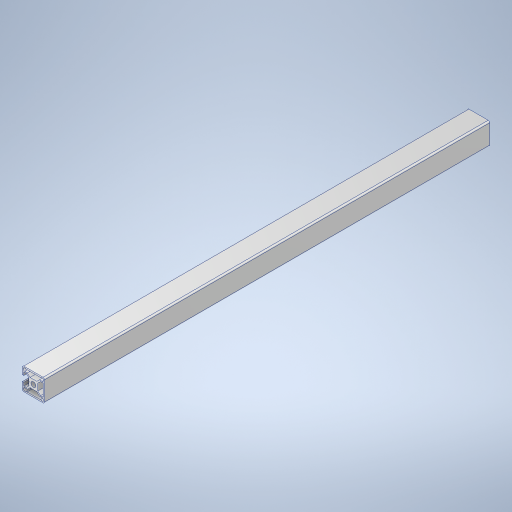
# Autodesk Inventor part: HFSC6-3030-600
Saved by Autodesk Inventor 2024 (Build 280153000, 153)
## iProperties
Category: PARTsolutions
Company: MISUMI
Created: 2024-12-02
Part Number: HFSC6-3030-600
Material: Aluminum 6061
Catalog Web Link: www.cadenas.de
Description: NEFSF6-3030, EFSF6-3030, EFSFB6-3030, HFSF6-3030, HFSFB6-3030, EFSH6-3030, HFSH6-3030, NEFST6-3030, EFST6-3030,  EFSTB6-3030, HFST6-3030, HFSTB6-3030, EFSC6-3030, HFSC6-3030-HFS6 Series Aluminum Extrusions 30 Square -1 Slot-
Vendor: MISUMI
Document SubType Name: Modeling
Designer: psAdmin
Manufacturer: MISUMI
Mass: 583.629 g
Surface Area: 2047.22 cm^2
Volume: 216.159 cm^3
Density: 2.7 g/cm^3
Appearance: Aluminum - Flat
PSOL_IDENT_0: {$CADENAS_DATA/23d-libs/misumi/metric/38_al_extrusions_blackets/6/hfsf6_3030.prj},748 {VTYP=3D},{NB=
PSOL_IDENT_1: HFSC6-3030-600},{LINA=HFSC6-3030-600},{NN=NEFSF6-3030, EFSF6-3030, EFSFB6-3030, HFSF6-3030, HFSFB6-3
PSOL_IDENT_2: 030, EFSH6-3030, HFSH6-3030, NEFST6-3030, EFST6-3030,  EFSTB6-3030, HFST6-3030, HFSTB6-3030, EFSC6-3
PSOL_IDENT_3: 030, HFSC6-3030},{DATE=31.01.2024 10:05:21},{GEOMDATE=26.07.2023 02:49:00},{VERSION=},{LINEID=190},{
PSOL_IDENT_4: WBVAR=L,ALT1,ALT2,ALT3,ALT4,ALT5,CP5,DL5,DR5,ALT6,ALT9,ALT10,ALT11,DD6SE,DD6,HP6,NHL6,DL6,NHR6,DR6,A
PSOL_IDENT_5: LT7,ALT8,NH9,AH,BH,CH,DH,EH,NH10,AV,BV,CV,DV,EV,NH11,AP,BP,CP,DP,EP,ALT12,ALT13,Z,NH12,XA,XB,XC,XD,X
PSOL_IDENT_6: E,NH13,YA,YB,YC,YD,YE,ALT14,HP14,DL14,DR14,ALT15,HP15,DL15,DR15,ALT16,HP16,DL16,DR16,ALT17,HQ17,JLP,
PSOL_IDENT_7: ALT20},{WBNUMERIC=L,DD6,NH9,AH,BH,CH,DH,EH,NH10,AV,BV,CV,DV,EV,NH11,AP,BP,CP,DP,EP,NH12,XA,XB,XC,XD,
PSOL_IDENT_8: XE,NH13,YA,YB,YC,YD,YE,HQ17,JLP}  {NB=HFSC6-3030-600},{LINA=HFSC6-3030-600},{KT=DUMMY},{PN=HFSC6-303
PSOL_IDENT_9: 0-600},{TPS=HFSC6-3030},{MAT=A6N01SS-T5 Aluminum Alloy},{ST=Clear Anodize},{FRMW=30},{FRMH=30},{FRD=
PSOL_IDENT_10: 6.8},{L=600.0},{MASS=0.97},{SA=361},{LX=2.99x10^4},{LY=3.24x10^4},{ALT1=},{M1=0},{DALT1=4.2},{DPL1=0
PSOL_IDENT_11: },{DPR1=0},{ALT1PN=},{ALT2=},{ALT2ALG= '','w/o End Tapping (Heli-Coil Insert)','LHP','with LHP (Tapp
PSOL_IDENT_12: ing on the Left (Heli-Coil Insert))','RHP','with RHP (Tapping on the Right (Heli-Coil Insert))','HPW'
PSOL_IDENT_13: ,'with HPW (Tapping on Both Ends (Heli-Coil Insert))' },{M2=0},{DP2=0},{ALT2PN=},{ALT3=},{ALT3ALG= ''
PSOL_IDENT_14: ,'w/o Tapping (Corner Section)','LSP','with LSP (Tapping (Corner Section))','RSP','with RSP (Tapping
PSOL_IDENT_15: (Corner Section))','SPW','with SPW (Tapping (Corner Section))' },{M3=0},{DP3=0},{ALT3PN=},{ALT4=},{
PSOL_IDENT_16: ALT4ALG= '', 'w/o SC (High Precision Cut)', 'SC', 'with SC (High Precision Cut)' },{ALT4PN=},{ALT5=}
PSOL_IDENT_17: ,{ALT5ALG= '','w/o 45 Degree Cut','1','with 45 Degree Cut' },{CP5=},{CP5ALG= '','N/A' },{DL5=},{DL5A
PSOL_IDENT_18: LG= '','N/A' },{DR5=},{DR5ALG= '','N/A' },{FRMLALT5=0},{FRMRALT5=0},{ALT5PN=},{ALT6=},{ALT6ALG= '','
PSOL_IDENT_19: w/o Fastening Location Wrench Access Hole Alterations','1','with Fastening Location Wrench Access Ho
PSOL_IDENT_20: le Alterations' },{ALT9=},{ALT9ALG= '','w/o Location Specified Wrench Access Hole Alteratons (Horizo
PSOL_IDENT_21: ntal)','1','with Location Specified Wrench Access Hole Alteratons (Horizontal)' },{ALT10=},{ALT10ALG=
PSOL_IDENT_22: '','w/o Location Specified Wrench Access Hole Alteratons (Vertical)','1','with Location Specified W
PSOL_IDENT_23: rench Access Hole Alteratons (Vertical)' },{ALT11=},{ALT11ALG= '','w/o Location Specified Wrench Acc
PSOL_IDENT_24: ess Hole Alteratons (Crisscross)','1','with Location Specified Wrench Access Hole Alteratons (Crissc
PSOL_IDENT_25: ross)' },{DD6SE=},{DD6SEALG= '','N/A' },{DD6=0},{DD6ALG=0},{HP6=},{HP6ALG= '','N/A' },{NHL6=},{NHL6A
PSOL_IDENT_26: LG= '','N/A' },{DL6=},{DL6ALG= '','N/A' },{NHR6=},{NHR6ALG= '','N/A' },{DR6=},{DR6ALG= '','N/A' },{D
PSOL_IDENT_27: D6PN=},{HL6=0},{HL6D=0},{HR6=0},{HR6D=0},{J6=0},{J6D=0},{K6=0},{K6D=0},{ALT7=},{ALT7ALG= '','N/A' },
PSOL_IDENT_28: {ALT8=},{ALT8ALG= '','N/A' },{ALT678PN=},{NH9=0},{NH9MAX=5},{NH9ALG=[0]},{AH=0.0},{AHMIN=7},{AHMAX=5
PSOL_IDENT_29: 95},{AHALG=[0]},{BH=0.0},{BHMIN=2},{BHMAX=597},{BHALG=[0]},{CH=0.0},{CHMIN=2},{CHMAX=599},{CHALG=[0]
PSOL_IDENT_30: },{DH=0.0},{DHMIN=2},{DHMAX=601},{DHALG=[0]},{EH=0.0},{EHMIN=2},{EHMAX=593},{EHALG=[0]},{NH10=0},{NH
PSOL_IDENT_31: 10MAX=5},{NH10ALG=[0]},{AV=0.0},{AVMIN=7},{AVMAX=595},{AVALG=[0]},{BV=0.0},{BVMIN=2},{BVMAX=597},{BV
PSOL_IDENT_32: ALG=[0]},{CV=0.0},{CVMIN=2},{CVMAX=599},{CVALG=[0]},{DV=0.0},{DVMIN=2},{DVMAX=601},{DVALG=[0]},{EV=0
PSOL_IDENT_33: .0},{EVMIN=2},{EVMAX=593},{EVALG=[0]},{NH11=0},{NH11MAX=5},{NH11ALG=[0]},{AP=0.0},{APMIN=7},{APMAX=5
PSOL_IDENT_34: 95},{APALG=[0]},{BP=0.0},{BPMIN=2},{BPMAX=597},{BPALG=[0]},{CP=0.0},{CPMIN=2},{CPMAX=599},{CPALG=[0]
PSOL_IDENT_35: },{DP=0.0},{DPMIN=2},{DPMAX=601},{DPALG=[0]},{EP=0.0},{EPMIN=2},{EPMAX=593},{EPALG=[0]},{ALT9PN=},{A
PSOL_IDENT_36: LT10PN=},{ALT11PN=},{ALT91011PN=},{ALT12=},{ALT12ALG= '' ,'N/A' },{ALT13=},{ALT13ALG= '','N/A' },{Z=
PSOL_IDENT_37: },{ZALG= '','N/A' },{DD12=0.0},{DD112=0.0},{NH12=0},{NH12MAX=5},{NH12ALG=[0]},{XA=0.0},{XAMIN=7},{XA
PSOL_IDENT_38: MAX=595},{XAALG=[0]},{XB=0.0},{XBMIN=2},{XBMAX=597},{XBALG=[0]},{XC=0.0},{XCMIN=2},{XCMAX=599},{XCAL
PSOL_IDENT_39: G=[0]},{XD=0.0},{XDMIN=2},{XDMAX=601},{XDALG=[0]},{XE=0.0},{XEMIN=2},{XEMAX=593},{XEALG=[0]},{NH13=0
PSOL_IDENT_40: },{NH13MAX=5},{NH13ALG=[0]},{YA=0.0},{YAMIN=7},{YAMAX=595},{YAALG=[0]},{YB=0.0},{YBMIN=2},{YBMAX=597
PSOL_IDENT_41: },{YBALG=[0]},{YC=0.0},{YCMIN=2},{YCMAX=599},{YCALG=[0]},{YD=0.0},{YDMIN=2},{YDMAX=601},{YDALG=[0]},
PSOL_IDENT_42: {YE=0.0},{YEMIN=2},{YEMAX=593},{YEALG=[0]},{ALT12PN=},{ALT13PN=},{ALT1213PN=},{ALT14=},{ALT14ALG= ''
PSOL_IDENT_43: ,'w/o D Type Hole Alteration','1','with D Type Hole Alteration' },{HP14=},{HP14ALG= '','N/A' },{DL14=
PSOL_IDENT_44: },{DL14ALG= '','N/A' },{DR14=},{DR14ALG= '','N/A' },{H14=0},{D14=0.0},{ALT14PN=},{ALT15=},{ALT15ALG=
PSOL_IDENT_45: '','N/A' },{HP15=},{HP15ALG= '','N/A' },{DL15=},{DL15ALG= '','N/A' },{DR15=},{DR15ALG= '','N/A' },{
PSOL_IDENT_46: H15=0},{D115=0.0},{D215=0.0},{ALT15PN=},{ALT16=},{ALT16ALG= '','w/o M Type Hole Alteration','1','wit
PSOL_IDENT_47: h M Type Hole Alteration' },{HP16=},{HP16ALG= '','N/A' },{DL16=},{DL16ALG= '','N/A' },{DR16=},{DR16A
PSOL_IDENT_48: LG= '','N/A' },{H116=0},{D16=0.0},{ALT16PN=},{ALT17=},{ALT17ALG= '','N/A' },{HQ17=0},{HQ17ALG=0},{JL
PSOL_IDENT_49: P=0},{JLPMIN=4.9},{JLPMAX=0},{JLPALG=[0]},{L17=0},{D17=0.0},{ALT17PN=},{ALT20=},{ALT20PN=},{ERRORALT
PSOL_IDENT_50: 01=OK},{ERRORALT02=OK},{ERRORALT03=OK},{ERRORALT05=OK},{ERRORALT06091=OK},{ERRORALT06092=OK},{ERRORA
PSOL_IDENT_51: LT06093=OK},{ERRORALT06094=OK},{ERRORALT06101=OK},{ERRORALT06102=OK},{ERRORALT06103=OK},{ERRORALT061
PSOL_IDENT_52: 04=OK},{ERRORALT06111=OK},{ERRORALT06112=OK},{ERRORALT06113=OK},{ERRORALT06114=OK},{ERRORALT06121=OK
PSOL_IDENT_53: },{ERRORALT06122=OK},{ERRORALT06123=OK},{ERRORALT06124=OK},{ERRORALT06131=OK},{ERRORALT06132=OK},{ER
PSOL_IDENT_54: RORALT06133=OK},{ERRORALT06134=OK},{ERRORALT0614=OK},{ERRORALT0615=OK},{ERRORALT0616=OK},{ERRORALT06
PSOL_IDENT_55: 171=OK},{ERRORALT06172=OK},{ERRORALT06173=OK},{ERRORALT0911=OK},{ERRORALT0913=OK},{ERRORALT0914=OK},
PSOL_IDENT_56: {ERRORALT0915=OK},{ERRORALT0916=OK},{ERRORALT0917=OK},{ERRORALT1011=OK},{ERRORALT1012=OK},{ERRORALT1
PSOL_IDENT_57: 014=OK},{ERRORALT1015=OK},{ERRORALT1016=OK},{ERRORALT1017=OK},{ERRORALT1112=OK},{ERRORALT1113=OK},{E
PSOL_IDENT_58: RRORALT1114=OK},{ERRORALT1115=OK},{ERRORALT1116=OK},{ERRORALT1117=OK},{ERRORALT1214=OK},{ERRORALT121
PSOL_IDENT_59: 5=OK},{ERRORALT1216=OK},{ERRORALT1217=OK},{ERRORALT1314=OK},{ERRORALT1315=OK},{ERRORALT1316=OK},{ERR
PSOL_IDENT_60: ORALT1317=OK},{ERRORALT1415=OK},{ERRORALT1416=OK},{ERRORALT1417=OK},{ERRORALT1516=OK},{ERRORALT1517=
PSOL_IDENT_61: OK},{ERRORALT1617=OK},{ERRORPN=},{IDM1=6.647},{IDM3=4.134},{TFW=2},{TFH=2.000}
NB: HFSC6-3030-600
NN: NEFSF6-3030, EFSF6-3030, EFSFB6-3030, HFSF6-3030, HFSFB6-3030, EFSH6-3030, HFSH6-3030, NEFST6-3030, EFST6-3030,  EFSTB6-3030, HFST6-3030, HFSTB6-3030, EFSC6-3030, HFSC6-3030
NT: HFS6 Series Aluminum Extrusions 30 Square -1 Slot-
NBSYN: $PN.
LINA: HFSC6-3030-600
CATALOG: Misumi
PN: HFSC6-3030-600
TPS: HFSC6-3030
MAT: A6N01SS-T5 Aluminum Alloy
ST: Clear Anodize
L: 600
MASS: 0.97
SA: 361
LX: 2.99x10^4
LY: 3.24x10^4
ALT1: w/o End Tapping
M1: 0
DPL1: 0
DPR1: 0
ALT2: w/o End Tapping (Heli-Coil Insert)
M2: 0
DP2: 0
ALT3: w/o Tapping (Corner Section)
M3: 0
DP3: 0
ALT4: w/o SC (High Precision Cut)
ALT5: w/o 45 Degree Cut
CP5: N/A
DL5: N/A
DR5: N/A
ALT6: w/o Fastening Location Wrench Access Hole Alterations
ALT9: w/o Location Specified Wrench Access Hole Alteratons (Horizontal)
ALT10: w/o Location Specified Wrench Access Hole Alteratons (Vertical)
ALT11: w/o Location Specified Wrench Access Hole Alteratons (Crisscross)
DD6SE: N/A
DD6: 0
HP6: N/A
NHL6: N/A
DL6: N/A
NHR6: N/A
DR6: N/A
HL6D: 0
HR6D: 0
J6D: 0
K6D: 0
ALT7: N/A
ALT8: N/A
NH9: 0
AH: 0
BH: 0
CH: 0
DH: 0
EH: 0
NH10: 0
AV: 0
BV: 0
CV: 0
DV: 0
EV: 0
NH11: 0
AP: 0
BP: 0
CP: 0
DP: 0
EP: 0
ALT12: N/A
ALT13: N/A
Z: N/A
DD12: 0
DD112: 0
NH12: 0
XA: 0
XB: 0
XC: 0
XD: 0
XE: 0
NH13: 0
YA: 0
YB: 0
YC: 0
YD: 0
YE: 0
ALT14: w/o D Type Hole Alteration
HP14: N/A
DL14: N/A
DR14: N/A
H14: 0
D14: 0
ALT15: N/A
HP15: N/A
DL15: N/A
DR15: N/A
H15: 0
D115: 0
D215: 0
ALT16: w/o M Type Hole Alteration
HP16: N/A
DL16: N/A
DR16: N/A
H116: 0
D16: 0
ALT17: N/A
HQ17: 0
JLP: 0
D17: 0
ALT20: w/o CW (End Face C Chamfering)
SUPPLIER: MISUMI
ARTICLENO: HFSC6-3030-600
BOMINFO: HFSC6-3030-600
CREATOR: CADENAS GmbH
Title: HFSC6-3030-600
Author: Cadenas PARTsolutions
Comments: HFS6 Series Aluminum Extrusions 30 Square -1 Slot-
Autodesk Inventor part; units mm, degrees
sketch "Sketch_122" plane through (0, 0, 0) normal (0, 0, 1) x (1, 0, 0)
  arc A0 (-15, -13) -> (-13, -15) centre (-13, -13) ccw
  line L0 (-13, -15) -> (13, -15)
  arc A1 (13, -15) -> (15, -13) centre (13, -13) ccw
  line L1 (15, -13) -> (15, 13)
  arc A2 (15, 13) -> (13, 15) centre (13, 13) ccw
  line L2 (13, 15) -> (-13, 15)
  arc A3 (-13, 15) -> (-15, 13) centre (-13, 13) ccw
  line L3 (-15, 13) -> (-15, 4)
  line L4 (-15, 4) -> (-13, 4)
  line L5 (-13, 4) -> (-13, 8.25)
  line L6 (-13, 8.25) -> (-9.6642, 8.25)
  line L7 (-9.6642, 8.25) -> (-6, 4.5858)
  line L8 (-6, 4.5858) -> (-6, 0.5196)
  line L9 (-6, 0.5196) -> (-5.7, 0)
  line L10 (-5.7, 0) -> (-6, -0.5196)
  line L11 (-6, -0.5196) -> (-6, -4.5858)
  line L12 (-6, -4.5858) -> (-9.6642, -8.25)
  line L13 (-9.6642, -8.25) -> (-13, -8.25)
  line L14 (-13, -8.25) -> (-13, -4)
  line L15 (-13, -4) -> (-15, -4)
  line L16 (-15, -4) -> (-15, -13)
  line L17 (6, -4.5858) -> (9.6642, -8.25)
  line L18 (9.6642, -8.25) -> (13, -8.25)
  line L19 (13, -8.25) -> (13, 8.25)
  line L20 (13, 8.25) -> (9.6642, 8.25)
  line L21 (9.6642, 8.25) -> (6, 4.5858)
  line L22 (6, 4.5858) -> (6, -4.5858)
  constraints: 46 end point, 8 point on circle, 4 centre point
extrude "Extrusion1" add sketch "Sketch_122" against normal blind 600
sketch "Sketch2" plane through (0, 0, -600) normal (0, 0, -1) x (-1, 0, 0)
  point P0 (0, 0)
hole "Hole1" at (0, 0, -600) direction (0, 0, 1) diameter 6.8 depth 600
sketch "Sketch_173" plane through (0, 0, 0) normal (0, 0, 1) x (1, 0, 0)
  arc A0 (-9.8177, 12.6944) -> (-11.625, 9.525) centre (-11.625, 11.625) ccw
  line L0 (-11.625, 9.525) -> (-8.1108, 9.525)
  line L1 (-8.1108, 9.525) -> (-4.5858, 6)
  line L2 (-4.5858, 6) -> (4.5858, 6)
  line L3 (4.5858, 6) -> (8.1108, 9.525)
  line L4 (8.1108, 9.525) -> (11.625, 9.525)
  arc A1 (11.625, 9.525) -> (9.8177, 12.6944) centre (11.625, 11.625) ccw
  arc A2 (8.7013, 13) -> (9.8177, 12.6944) centre (9.3013, 13) ccw
  line L5 (8.7013, 13) -> (-8.7013, 13)
  arc A3 (-9.8177, 12.6944) -> (-8.7013, 13) centre (-9.3013, 13) ccw
  constraints: 12 end point, 8 point on circle, 4 centre point
extrude "Extrusion2" cut sketch "Sketch_173" against normal blind 600
sketch "Sketch_174" plane through (0, 0, 0) normal (0, 0, 1) x (1, 0, 0)
  arc A0 (-11.625, -9.525) -> (-9.8177, -12.6944) centre (-11.625, -11.625) ccw
  arc A1 (-8.7013, -13) -> (-9.8177, -12.6944) centre (-9.3013, -13) ccw
  line L0 (-8.7013, -13) -> (8.7013, -13)
  arc A2 (9.8177, -12.6944) -> (8.7013, -13) centre (9.3013, -13) ccw
  arc A3 (9.8177, -12.6944) -> (11.625, -9.525) centre (11.625, -11.625) ccw
  line L1 (11.625, -9.525) -> (8.1108, -9.525)
  line L2 (8.1108, -9.525) -> (4.5858, -6)
  line L3 (4.5858, -6) -> (-4.5858, -6)
  line L4 (-4.5858, -6) -> (-8.1108, -9.525)
  line L5 (-8.1108, -9.525) -> (-11.625, -9.525)
  constraints: 12 end point, 8 point on circle, 4 centre point
extrude "Extrusion3" cut sketch "Sketch_174" against normal blind 600
ref_plane "C1_XY" through (0, 0, 0) normal (0, 0, 1) x (1, 0, 0)
ref_plane "C1_YZ" through (0, 0, 0) normal (1, 0, 0) x (0, 1, 0)
ref_plane "C1_ZX" through (0, 0, 0) normal (0, 1, 0) x (0, 0, 1)
ref_plane "to_frame_cap1_XY" through (0, 0, 0) normal (0, 0, 1) x (1, 0, 0)
ref_plane "to_frame_cap1_YZ" through (0, 0, 0) normal (1, 0, 0) x (0, 1, 0)
ref_plane "to_frame_cap1_ZX" through (0, 0, 0) normal (0, 1, 0) x (0, 0, 1)
ref_plane "to_frame_cap2_XY" through (0, 0, -600) normal (0, 0, -1) x (1, 0, 0)
ref_plane "to_frame_cap2_YZ" through (0, 0, -600) normal (1, 0, 0) x (0, -1, 0)
ref_plane "to_frame_cap2_ZX" through (0, 0, -600) normal (0, -1, 0) x (0, 0, -1)
thread "Thread1" size "M8x1.25" class "6H" standard "ANSI Metric M Profile" length 10
thread "Thread2" size "M7x1" class "6H" standard "ANSI Metric M Profile" length 10
body "Solid1"
